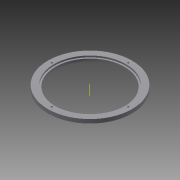
# Autodesk Inventor part: Mirror Support
Saved by Autodesk Inventor 2015 (Build 190159000, 159)
## iProperties
Created: 2014-07-17
Part Number: Mirror Support
Material: Generic
Document SubType Name: Modeling
Designer: I Rabey
Density: 1 g/cm^3
Appearance: Default
Author: I Rabey
Autodesk Inventor part; units mm, degrees
ref_plane "YZ Plane" through (0, 0, 0) normal (1, 0, 0) x (0, 1, 0)
ref_plane "XZ Plane" through (0, 0, 0) normal (0, 1, 0) x (-1, 0, 0)
ref_plane "XY Plane" through (0, 0, 0) normal (0, 0, 1) x (1, 0, 0)
sketch "Sketch1" plane through (0, 0, 0) normal (0, 1, 0) x (-1, 0, 0)
  circle A0 centre (0, 0) radius 45
  circle A1 centre (0, 0) radius 55
  dimension "d0" = 90
  dimension "d1" = 110
  constraints: 2 centre point, 2 coincident
  measures "d0" diameter of A0
  measures "d1" diameter of A1
extrude "Extrusion1" add sketch "Sketch1" along normal blind 5
sketch "Sketch2" plane through (0, 5, 0) normal (0, 1, 0) x (1, 0, 0)
  circle A0 centre (0, 0) radius 45
  circle A1 centre (0, 0) radius 47
  dimension "d4" = 90
  dimension "d5" = 94
  constraints: 2 centre point, 2 coincident
  measures "d4" diameter of A0
  measures "d5" diameter of A1
extrude "Extrusion2" cut sketch "Sketch2" against normal blind 2
sketch "Sketch3" plane through (0, 5, 0) normal (0, 1, 0) x (1, 0, 0)
  circle A0 centre (0, -50) radius 1
  circle A1 centre (0, 0) radius 55 projected
  dimension "d8" = 2
  dimension "d9" = 50
  constraints: 1 centre point
  measures "d8" diameter of A0
  measures "d9" distance of A1.centre A0.centre
hole "Hole1" at (0, 5, 50) direction (0, -1, 0) diameter 2 end through all
sketch "Sketch4" plane through (0, 5, 0) normal (0, 1, 0) x (1, 0, 0)
  circle A0 centre (-50, 0) radius 1
  point P0 (0, 0)
  dimension "d17" = 2
  dimension "d18" = 50
  constraints: 1 centre point
  measures "d17" diameter of A0
  measures "d18" distance of point (0, 0) A0.centre
sketch "Sketch5" plane through (0, 5, 0) normal (0, 1, 0) x (1, 0, 0)
  circle A0 centre (0, 50) radius 1
  point P0 (0, 0)
  dimension "d19" = 2
  dimension "d20" = 50
  constraints: 1 centre point
  measures "d19" diameter of A0
  measures "d20" distance of point (0, 0) A0.centre
sketch "Sketch6" plane through (0, 5, 0) normal (0, 1, 0) x (1, 0, 0)
  circle A0 centre (50, 0) radius 1
  point P0 (0, 0)
  dimension "d21" = 2
  dimension "d22" = 50
  constraints: 1 centre point
  measures "d21" diameter of A0
  measures "d22" distance of point (0, 0) A0.centre
hole "Hole2" at (-50, 5, 0) direction (0, -1, 0) diameter 2 end through all
hole "Hole3" at (0, 5, -50) direction (0, -1, 0) diameter 2 end through all
hole "Hole4" at (50, 5, 0) direction (0, -1, 0) diameter 2 end through all
thread "Thread1" size "2-56 UNC" class "2B" standard "ANSI Unified Screw Threads" full length
thread "Thread2" size "2-56 UNC" class "2B" standard "ANSI Unified Screw Threads" full length
thread "Thread3" size "2-56 UNC" class "2B" standard "ANSI Unified Screw Threads" full length
thread "Thread4" size "2-56 UNC" class "2B" standard "ANSI Unified Screw Threads" full length
body "Solid1"
